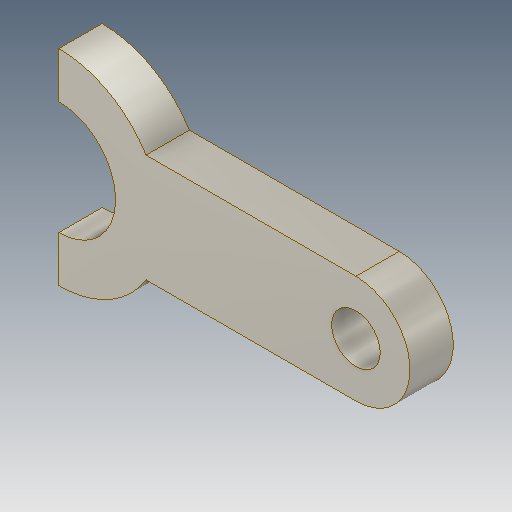
# Autodesk Inventor part: garfo-1
Saved by Autodesk Inventor 2017 (Build 210142000, 142)
## iProperties
Created: 2018-05-30
Part Number: garfo-1
Material: Generic
Document SubType Name: Modeling
Designer: Luiz Gustavo
Density: 1 g/cm^3
Appearance: Titanium
Mass: 1.2257 g
Surface Area: 10.6484 cm^2
Volume: 1.2257 cm^3
Author: Luiz Gustavo
Autodesk Inventor part; units mm, degrees
ref_plane "YZ Plane" through (0, 0, 0) normal (1, 0, 0) x (0, 1, 0)
ref_plane "XZ Plane" through (0, 0, 0) normal (0, 1, 0) x (-1, 0, 0)
ref_plane "XY Plane" through (0, 0, 0) normal (0, 0, 1) x (1, 0, 0)
sketch "Sketch1" plane through (0, 0, 0) normal (0, 0, 1) x (1, 0, 0)
  arc A0 (0, -5.25) -> (0, 5.25) centre (0, 0) ccw
  arc A1 (8.0777, 5) -> (0, 9.5) centre (0, 0) ccw
  line L0 (0, 0) -> (27.5, 0) construction
  arc A2 (27.5, 5) -> (27.5, -5) centre (27.5, 0) ccw construction
  line L1 (0, 9.5) -> (0, 5.25)
  line L2 (27.5, 5) -> (8.0777, 5)
  line L3 (27.5, -5) -> (8.0777, -5)
  arc A3 (27.5, -5) -> (27.5, 5) centre (27.5, 0) ccw
  circle A4 centre (27.5, 0) radius 2.25
  arc A5 (0, 9.5) -> (0, -9.5) centre (0, 0) ccw construction
  arc A6 (0, -9.5) -> (8.0777, -5) centre (0, 0) ccw
  arc A7 (0, 5.25) -> (0, -5.25) centre (0, 0) ccw construction
  line L4 (0, 5.25) -> (0, -5.25) construction
  line L5 (0, -5.25) -> (0, -9.5)
  dimension "d2" = 10
  dimension "d4" = 4.5
  dimension "d5" = 5.25
  dimension "d6" = 9.5
  dimension "d7" = 27.5
  constraints: 15 point on circle, 12 end point, 8 centre point, 5 coincident, 3 horizontal, 3 vertical, 2 tangent, 1 midpoint, 1 point on line
  measures "d2" diameter of A2
  measures "d4" diameter of A4
  measures "d5" radius of A0
  measures "d6" radius of A1
  measures "d7" distance of L0.start L0.end
extrude "Extrusion1" add sketch "Sketch1" along normal mid plane 4
body "Solid1"
